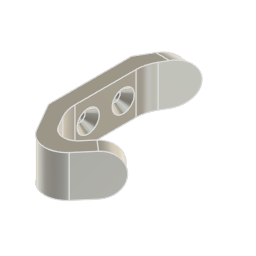
ElbowBracket (Autodesk Fusion 360 design; units mm, degrees)
Autodesk Fusion 360 part; units mm, degrees
note: some values were not read from the file. Set by a fixed rule: which sketch regions a step uses.
sketch "Sketch1" plane through (0, 0, 0) normal (0, 0, 1) x (1, 0, 0)
  line L0 (0, 30) -> (0, 0)
  line L1 (0, 0) -> (5.8903, -10.2022)
  line L2 (18.899, -11.401) -> (28.6467, 0)
  line L3 (5, 30) -> (5, 1.3397)
  line L4 (5, 1.3397) -> (8.8062, -5.2528)
  line L5 (16.9367, -6.002) -> (24.8463, 3.2492)
  line L6 (24.8463, 3.2492) -> (28.6467, 0)
  arc A0 (8.8062, -5.2528) -> (16.9367, -6.002) centre (13.1363, -2.7528) ccw
  arc A1 (5.8903, -10.2022) -> (18.899, -11.401) centre (12.8185, -6.2022) ccw
  line L7 (0, 30) -> (7.5, 42.9904)
  line L8 (5, 30) -> (12.5581, 42.9567)
  line L9 (7.5, 42.9904) -> (12.5581, 42.9567)
  point P0 (11.547, -20)
  dimension "d1" = 30
  dimension "d2" = 20
  dimension "d3" = 150
  dimension "d5" = 20
  dimension "d6" = 5
  dimension "d7" = 8
  dimension "d21" = 15
  dimension "d22" = 150
  constraint vertical L0
  constraint coincident L0.end L1.start
  constraint perpendicular L2 L6
  constraint tangent L5 A0
  constraint tangent L4 A0
  constraint coincident P0 L1
  constraint coincident P0 L2
  constraint tangent L1 A1
  constraint tangent L2 A1
  constraint equal L2 L7
  constraint equal L7 L8
  measures "d1" distance of L0.start L0.end
  measures "d2" vertical distance of L0.end P0
  measures "d3" angle of L0 L1
  measures "d5" vertical distance of P0 L2.end
  measures "d6" radius of A0
  measures "d7" radius of A1
  measures "d21" distance of L0.start L7.end
  measures "d22" angle of L0 L7
extrude "Extrude1" add sketch "Sketch1" along normal blind 15
sketch "Sketch2" plane through (5, 0, 0) normal (1, 0, 0) x (0, 1, 0)
  line L0 (1.3397, 0) -> (30, 0)
  line L1 (30, 15) -> (1.3397, 15)
  line L2 (1.3397, 15) -> (1.3397, 0)
  line L3 (15.6699, 15) -> (15.6699, 0) construction
  line L4 (30, 7.5) -> (1.3397, 7.5) construction
  circle A0 centre (9.3397, 7.5) radius 4
  circle A1 centre (22, 7.5) radius 4
  line L5 (30, 0) -> (30, 15)
  dimension "d10" = 8
  dimension "d11" = 8
  constraint midpoint L1 L3.start
  constraint midpoint L0 L3.end
  constraint midpoint L2 L4.end
  constraint coincident L4 A0.centre
  constraint symmetric L3 A0 A1
  measures "d10" diameter of A0
  measures "d11" distance of L4.end A0.centre
extrude "Extrude2" cut sketch "Sketch2" against normal blind 3 draft -35 contours A0 | A1
extrude "Extrude3" cut 2 faces at (2, 8.7693, 7.7747) (2, 21.4769, 7.1433) along direction (-1, 0, 0) through all
fillet "Fillet1" radius 7.5 2 edges at (26.7465, 1.6246, 15) (26.7465, 1.6246, 0)
fillet "Fillet2" [no effect]
fillet "Fillet3" radius 12 1 edges at (5, 1.3397, 7.5)
fillet "Fillet4" radius 7.5 2 edges at (10.029, 42.9735, 15) (10.029, 42.9735, 0)
fillet "Fillet5" radius 12.5 1 edges at (5, 30, 7.5)
